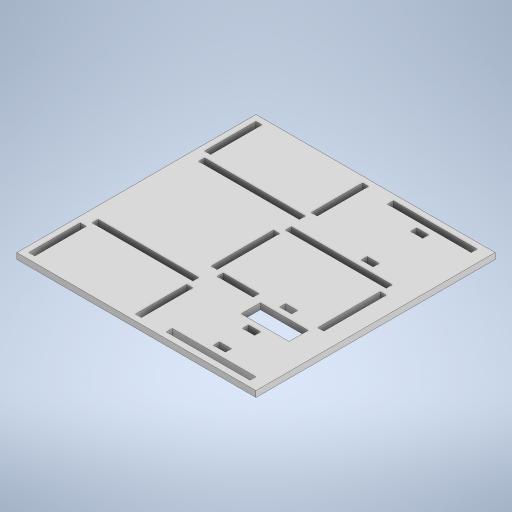
# Autodesk Inventor part: base
Saved by Autodesk Inventor 2023 (Build 270158000, 158)
## iProperties
Created: 2023-11-13
Part Number: base
Material: Generic
Document SubType Name: Modeling
Designer: Nate
Density: 1 g/cm^3
Appearance: Default
Author: Nate
Autodesk Inventor part; units mm, degrees
ref_plane "YZ Plane" through (0, 0, 0) normal (1, 0, 0) x (0, 1, 0)
ref_plane "XZ Plane" through (0, 0, 0) normal (0, 1, 0) x (-1, 0, 0)
ref_plane "XY Plane" through (0, 0, 0) normal (0, 0, 1) x (1, 0, 0)
sketch "Sketch1" plane through (0, 0, 0) normal (0, 1, 0) x (-1, 0, 0)
  line L0 (0, 0) -> (127, 0)
  line L1 (127, 0) -> (127, -127)
  line L2 (127, -127) -> (0, -127)
  line L3 (0, -127) -> (0, 0)
  line L4 (123.825, 0) -> (127, 0)
  line L5 (127, 0) -> (127, -33.615)
  line L6 (127, -33.615) -> (123.825, -33.615)
  line L7 (123.825, -33.615) -> (123.825, 0)
  line L8 (123.825, -33.615) -> (70.363, -33.615)
  line L9 (70.363, -33.615) -> (70.363, -36.79)
  line L10 (70.363, -36.79) -> (127, -36.79)
  line L11 (70.363, -36.79) -> (67.188, -36.79)
  line L12 (67.188, -36.79) -> (67.188, 0)
  line L13 (67.188, 0) -> (70.363, 0)
  line L14 (70.363, 0) -> (70.363, -36.79)
  line L15 (69.1283, -45.3517) -> (43.7283, -45.3517)
  line L16 (43.7283, -45.3517) -> (43.7283, -42.1767)
  line L17 (43.7283, -42.1767) -> (69.1283, -42.1767)
  line L18 (69.1283, -42.1767) -> (69.1283, -45.3517)
  line L19 (69.1283, -42.1767) -> (72.3033, -42.1767)
  line L20 (72.3033, -42.1767) -> (72.3033, -84.8107)
  line L21 (72.3033, -84.8107) -> (69.1283, -84.8107)
  line L22 (69.1283, -84.8107) -> (69.1283, -42.1767)
  line L23 (69.1283, -84.8107) -> (12.4863, -84.8107)
  line L24 (12.4863, -84.8107) -> (12.4863, -81.6357)
  line L25 (12.4863, -81.6357) -> (69.1283, -81.6357)
  line L26 (69.1283, -81.6357) -> (69.1283, -84.8107)
  line L27 (12.4863, -81.6357) -> (15.6613, -81.6357)
  line L28 (15.6613, -81.6357) -> (15.6613, -42.1767)
  line L29 (15.6613, -42.1767) -> (12.4863, -42.1767)
  line L30 (12.4863, -42.1767) -> (12.4863, -81.6357)
  line L31 (127, -90.21) -> (67.188, -90.21)
  line L32 (67.188, -90.21) -> (67.188, -93.385)
  line L33 (67.188, -93.385) -> (127, -93.385)
  line L34 (127, -93.385) -> (127, -90.21)
  line L35 (127, -93.385) -> (123.825, -93.385)
  line L36 (123.825, -93.385) -> (123.825, -127)
  line L37 (123.825, -127) -> (127, -127)
  line L38 (127, -127) -> (127, -93.385)
  line L39 (25.4, 0) -> (6.35, 0)
  line L40 (25.4, -127) -> (6.35, -127)
  line L41 (67.188, -90.21) -> (70.363, -90.21)
  line L42 (70.363, -90.21) -> (70.363, -127)
  line L43 (70.363, -127) -> (67.188, -127)
  line L44 (67.188, -127) -> (67.188, -90.21)
  line L45 (67.188, -3.175) -> (70.363, -3.175)
  line L46 (70.363, -3.175) -> (70.363, -33.615)
  line L47 (70.363, -33.615) -> (67.188, -33.615)
  line L48 (67.188, -33.615) -> (67.188, -3.175)
  line L49 (73.538, -33.615) -> (123.825, -33.615)
  line L50 (123.825, -33.615) -> (123.825, -36.79)
  line L51 (123.825, -36.79) -> (73.538, -36.79)
  line L52 (127, -3.175) -> (123.825, -3.175)
  line L53 (123.825, -3.175) -> (123.825, -30.44)
  line L54 (123.825, -30.44) -> (127, -30.44)
  line L55 (127, -30.44) -> (127, -3.175)
  line L56 (123.825, -90.21) -> (81.7068, -90.21)
  line L57 (81.7068, -93.385) -> (123.825, -93.385)
  line L58 (123.825, -93.385) -> (123.825, -90.21)
  line L59 (123.825, -96.56) -> (127, -96.56)
  line L60 (127, -96.56) -> (127, -123.825)
  line L61 (127, -123.825) -> (123.825, -123.825)
  line L62 (123.825, -123.825) -> (123.825, -96.56)
  line L63 (70.363, -96.56) -> (67.188, -96.56)
  line L64 (67.188, -96.56) -> (67.188, -123.825)
  line L65 (67.188, -123.825) -> (70.363, -123.825)
  line L66 (70.363, -123.825) -> (70.363, -96.56)
  line L67 (70.363, -30.44) -> (67.188, -30.44)
  line L68 (72.3033, -45.3517) -> (69.1283, -45.3517)
  line L69 (69.1283, -45.3517) -> (69.1283, -81.6357)
  line L70 (69.1283, -81.6357) -> (72.3033, -81.6357)
  line L71 (72.3033, -81.6357) -> (72.3033, -45.3517)
  line L72 (65.9533, -42.1767) -> (46.9033, -42.1767)
  line L73 (46.9033, -42.1767) -> (46.9033, -45.3517)
  line L74 (46.9033, -45.3517) -> (65.9533, -45.3517)
  line L75 (65.9533, -45.3517) -> (65.9533, -42.1767)
  line L76 (60.0198, -81.6357) -> (15.6613, -81.6357)
  line L77 (15.6613, -81.6357) -> (15.6613, -84.8107)
  line L78 (15.6613, -84.8107) -> (60.0198, -84.8107)
  line L79 (15.6613, -45.3517) -> (12.4863, -45.3517)
  line L80 (12.4863, -45.3517) -> (12.4863, -78.4607)
  line L81 (12.4863, -78.4607) -> (15.6613, -78.4607)
  line L82 (15.6613, -78.4607) -> (15.6613, -45.3517)
  line L83 (72.3033, -78.4607) -> (69.1283, -78.4607)
  line L84 (22.225, 0) -> (9.525, 0)
  line L85 (9.525, -127) -> (22.225, -127)
  line L86 (57.15, -3.175) -> (6.35, -3.175)
  line L87 (6.35, -3.175) -> (6.35, -6.35)
  line L88 (6.35, -6.35) -> (57.15, -6.35)
  line L89 (57.15, -6.35) -> (57.15, -3.175)
  line L90 (53.975, -3.175) -> (9.525, -3.175)
  line L91 (9.525, -3.175) -> (9.525, -6.35)
  line L92 (9.525, -6.35) -> (53.975, -6.35)
  line L93 (53.975, -6.35) -> (53.975, -3.175)
  line L94 (127, 0) -> (130.175, 0)
  line L95 (130.175, 0) -> (130.175, -127)
  line L96 (130.175, -127) -> (127, -127)
  line L97 (127, -127) -> (127, 0)
  line L98 (3.175, 0) -> (0, 0)
  line L99 (0, 0) -> (0, -127)
  line L100 (0, -127) -> (3.175, -127)
  line L101 (3.175, -127) -> (3.175, 0)
  line L102 (57.15, -120.65) -> (6.35, -120.65)
  line L103 (6.35, -120.65) -> (6.35, -123.825)
  line L104 (6.35, -123.825) -> (57.15, -123.825)
  line L105 (57.15, -123.825) -> (57.15, -120.65)
  line L106 (53.975, -120.65) -> (9.525, -120.65)
  line L107 (9.525, -120.65) -> (9.525, -123.825)
  line L108 (9.525, -123.825) -> (53.975, -123.825)
  line L109 (53.975, -123.825) -> (53.975, -120.65)
  line L110 (42.3948, -31.3817) -> (16.9948, -31.3817)
  line L111 (16.9948, -31.3817) -> (16.9948, -41.5417)
  line L112 (16.9948, -41.5417) -> (42.3948, -41.5417)
  line L113 (42.3948, -41.5417) -> (42.3948, -31.3817)
  line L114 (35.306, -9.525) -> (28.956, -9.525)
  line L115 (28.956, -9.525) -> (28.956, -12.7)
  line L116 (28.956, -12.7) -> (35.306, -12.7)
  line L117 (35.306, -12.7) -> (35.306, -9.525)
  line L118 (35.306, -25.0317) -> (28.956, -25.0317)
  line L119 (28.956, -25.0317) -> (28.956, -28.2067)
  line L120 (28.956, -28.2067) -> (35.306, -28.2067)
  line L121 (35.306, -28.2067) -> (35.306, -25.0317)
  line L122 (35.306, -44.7167) -> (28.956, -44.7167)
  line L123 (28.956, -44.7167) -> (28.956, -47.8917)
  line L124 (28.956, -47.8917) -> (35.306, -47.8917)
  line L125 (35.306, -47.8917) -> (35.306, -44.7167)
  line L126 (35.306, -87.9857) -> (28.956, -87.9857)
  line L127 (28.956, -87.9857) -> (28.956, -91.1607)
  line L128 (28.956, -91.1607) -> (35.306, -91.1607)
  line L129 (35.306, -91.1607) -> (35.306, -87.9857)
  line L130 (35.306, -114.3) -> (28.956, -114.3)
  line L131 (28.956, -114.3) -> (28.956, -117.475)
  line L132 (28.956, -117.475) -> (35.306, -117.475)
  line L133 (35.306, -117.475) -> (35.306, -114.3)
  point P0 (97.094, -33.615)
  point P1 (123.825, -110.1925)
  point P2 (123.825, -16.8075)
  point P3 (43.7283, -43.7642)
  point P4 (56.4283, -42.1767)
  point P5 (125.4125, 0)
  point P6 (125.4125, -3.175)
  point P7 (125.4125, -33.615)
  point P8 (70.363, -35.2025)
  point P9 (68.7755, -36.79)
  point P10 (68.7755, -33.615)
  point P11 (68.7755, 0)
  point P12 (68.7755, -3.175)
  point P13 (68.7755, -127)
  point P14 (68.7755, -123.825)
  point P15 (69.1283, -43.7642)
  point P16 (46.9033, -43.7642)
  point P17 (70.7158, -42.1767)
  point P18 (12.4863, -83.2232)
  point P19 (14.0738, -81.6357)
  point P20 (14.0738, -78.4607)
  point P21 (14.0738, -42.1767)
  point P22 (14.0738, -45.3517)
  point P23 (70.363, -93.385)
  point P24 (70.363, -30.44)
  point P25 (127, -96.56)
  point P26 (127, -30.44)
  point P27 (123.825, -33.615)
  point P28 (46.9033, -42.1767)
  point P29 (67.188, -96.56)
  point P30 (53.975, -4.7625)
  point P31 (53.975, -122.2375)
  point P32 (6.35, -122.2375)
  point P33 (15.875, -127)
  point P34 (127, -93.385)
  point P35 (53.975, -6.35)
  point P36 (32.131, -91.1607)
  dimension "d0" = 127
  dimension "d2" = 127
  dimension "d5" = 33.615
  dimension "d6" = 33.615
  dimension "d7" = 53.462
  dimension "d8" = 53.462
  dimension "d9" = 3.175
  dimension "d10" = 3.175
  dimension "d11" = 3.175
  dimension "d12" = 3.175
  dimension "d13" = 3.175
  dimension "d14" = 3.175
  dimension "d19" = 36.284
  dimension "d20" = 25.4
  dimension "d21" = 3.175
  dimension "d22" = 3.175
  dimension "d23" = 3.175
  dimension "d24" = 3.175
  dimension "d25" = 53.467
  dimension "d27" = 42.1767
  dimension "d28" = 3.175
  dimension "d29" = 3.175
  dimension "d30" = 3.175
  dimension "d32" = 3.175
  dimension "d33" = 3.175
  dimension "d34" = 3.175
  dimension "d35" = 3.175
  dimension "d36" = 3.175
  dimension "d37" = 3.175
  dimension "d38" = 3.175
  dimension "d39" = 3.175
  dimension "d40" = 3.175
  dimension "d41" = 3.175
  dimension "d42" = 3.175
  dimension "d43" = 3.175
  dimension "d44" = 3.175
  dimension "d45" = 3.175
  dimension "d46" = 3.175
  dimension "d51" = 3.175
  dimension "d52" = 3.175
  dimension "d53" = 3.175
  dimension "d54" = 50.8
  dimension "d55" = 3.175
  dimension "d56" = 6.35
  dimension "d57" = 3.175
  dimension "d58" = 3.175
  dimension "d59" = 3.175
  dimension "d60" = 3.175
  dimension "d61" = 3.175
  dimension "d62" = 50.8
  dimension "d63" = 6.35
  dimension "d64" = 3.175
  dimension "d65" = 9.3112
  dimension "d66" = 25.4
  dimension "d67" = 10.16
  dimension "d68" = 3.81
  dimension "d69" = 1.3335
  dimension "d70" = 6.35
  dimension "d71" = 3.175
  dimension "d72" = 3.175
  dimension "d73" = 6.35
  dimension "d74" = 3.175
  dimension "d75" = 3.175
  dimension "d76" = 6.35
  constraints: 268 end point, 62 parallel, 42 point on line, 36 horizontal, 34 perpendicular, 28 midpoint
  measures "d0" distance between parallel lines of L2 L0
  measures "d2" distance between parallel lines of L1 L3
  measures "d5" distance from line of point (97.094, -33.615) L0
  measures "d6" distance between parallel lines of L2 L33
  measures "d7" distance from line of point (123.825, -110.192) L42
  measures "d8" distance from line of L14 point (123.825, -16.808)
  measures "d9" distance between parallel lines of L5 L7
  measures "d10" distance between parallel lines of L1 L36
  measures "d11" distance between parallel lines of L42 L44
  measures "d12" distance between parallel lines of L14 L12
  measures "d13" distance between parallel lines of L10 L8
  measures "d14" distance between parallel lines of L33 L31
  measures "d19" distance between parallel lines of L25 L15
  measures "d20" distance from line of L22 point (43.728, -43.764)
  measures "d21" distance between parallel lines of L22 L20
  measures "d22" distance between parallel lines of L23 L25
  measures "d23" distance between parallel lines of L30 L28
  measures "d24" distance from line of L15 point (56.428, -42.177)
  measures "d25" distance between parallel lines of L22 L28
  measures "d27" distance between parallel lines of L17 L0
  measures "d28" distance of point (125.412, 0) point (125.413, -3.175)
  measures "d29" vertical distance of point (125.413, -33.615) L54.end
  measures "d30" distance between parallel lines of L1 L50
  measures "d32" distance of point (68.775, -36.79) point (68.775, -33.615)
  measures "d33" distance of point (68.775, 0) point (68.775, -3.175)
  measures "d34" distance between parallel lines of L47 L67
  measures "d35" distance between parallel lines of L33 L63
  measures "d36" distance of point (68.775, -127) point (68.775, -123.825)
  measures "d37" distance between parallel lines of L1 L58
  measures "d38" distance between parallel lines of L59 L35
  measures "d39" distance from line of point (69.128, -43.764) L75
  measures "d40" distance from line of L16 point (46.903, -43.764)
  measures "d41" distance from line of point (70.716, -42.177) L68
  measures "d42" distance between parallel lines of L21 L70
  measures "d43" distance between parallel lines of L70 L83
  measures "d44" distance from line of point (12.486, -83.223) L77
  measures "d45" distance of point (14.074, -81.636) point (14.074, -78.461)
  measures "d46" distance of point (14.074, -42.177) point (14.074, -45.352)
  measures "d51" distance from line of L89 point (53.975, -4.762)
  measures "d52" distance between parallel lines of L87 L91
  measures "d53" distance between parallel lines of L88 L86
  measures "d54" distance from line of L89 L87.end
  measures "d55" distance between parallel lines of L90 L0
  measures "d56" distance between parallel lines of L3 L87
  measures "d57" distance between parallel lines of L95 L97
  measures "d58" distance between parallel lines of L101 L99
  measures "d59" distance from line of L105 point (53.975, -122.237)
  measures "d60" distance between parallel lines of L103 L107
  measures "d61" distance between parallel lines of L104 L102
  measures "d62" distance from line of L105 L104.start
  measures "d63" distance from line of point (6.35, -122.237) L3
  measures "d64" distance from line of point (15.875, -127) L108
  measures "d65" distance between parallel lines of L101 L80
  measures "d66" distance of L112.end L111.end
  measures "d67" distance between parallel lines of L112 L110
  measures "d68" distance between parallel lines of L15 L112
  measures "d69" distance between parallel lines of L16 L113
  measures "d70" distance of L116.end L115.end
  measures "d71" distance of L115.end L114.end
  measures "d72" distance between parallel lines of L88 L114
  measures "d73" distance of L120.end L119.end
  measures "d74" distance of L119.end L118.end
  measures "d75" distance between parallel lines of L110 L120
  measures "d76" distance of L124.end L123.end
extrude "Extrusion1" add sketch "Sketch1" along normal blind 3.175 contours L0 L12 L11 L10 L1 L31 L32 L44 L2 L101 | L0 L14 L45 L12 | L0 L7 L8 L14 | L44 L65 L42 L2 | L0 L1 L52 L7 | L67 L14 L47 L12 | L42 L33 L36 L2 | L94 L95 L96 L1 | L47 L9 L11 L12 | L36 L61 L1 L2 | L44 L33 L42 L63 | L54 L1 L6 L7 | L32 L31 L42 L33 | L6 L1 L10 L50 | L36 L33 L1 L59 | L58 L31 L1 L33 | L15 L75 L17 L18 | L18 L19 L20 L68 | L83 L20 L70 L22 | L15 L16 L17 L73 | L70 L20 L21 L22 | L77 L23 L24 L25 | L25 L30 L81 L28 | L79 L30 L29 L28 | L89 L88 L93 L86 | L91 L88 L87 L86 | L105 L104 L109 L102 | L107 L104 L103 L102
equation "\"d3\" = d41"
body "Solid1"
